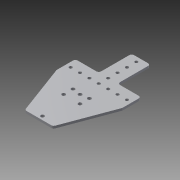
# Autodesk Inventor part: Roller Pneumatic Back Connector (Custom)
Saved by Autodesk Inventor 2014 (Build 180170000, 170)
## iProperties
Created: 2014-01-06
Part Number: Roller Pneumatic Back Connector (Custom)
Material: Aluminum 6061
Document SubType Name: Modeling
Designer: Andrew Toennies
Density: 2.71 g/cm^3
Appearance: Aluminum - Flat
Mass: 64.1686 g
Surface Area: 169.384 cm^2
Volume: 23.6785 cm^3
Author: Andrew Toennies
Autodesk Inventor part; units mm, degrees
ref_plane "YZ Plane" through (0, 0, 0) normal (1, 0, 0) x (0, 1, 0)
ref_plane "XZ Plane" through (0, 0, 0) normal (0, 1, 0) x (-1, 0, 0)
ref_plane "XY Plane" through (0, 0, 0) normal (0, 0, 1) x (1, 0, 0)
sketch "Sketch1" plane through (0, 0, 0) normal (0, 1, 0) x (-1, 0, 0)
  circle A0 centre (0, 0) radius 2.413
  circle A1 centre (0, 50.8) radius 2.413
  line L0 (0, 50.8) -> (0, 0) construction
  circle A2 centre (11.049, 11.1125) radius 2.413
  circle A3 centre (11.049, -1.5875) radius 2.413
  circle A4 centre (-11.049, -1.5875) radius 2.413
  circle A5 centre (-11.049, 11.1125) radius 2.413
  line L1 (-11.049, -1.5875) -> (-11.049, 11.1125) construction
  line L2 (-11.049, 11.1125) -> (11.049, 11.1125) construction
  line L3 (19.05, 55.5625) -> (-19.05, 55.5625)
  line L4 (-44.45, -12.7) -> (-44.45, -38.1)
  line L5 (-44.45, -38.1) -> (-15.875, -38.1)
  line L6 (-12.7, -41.275) -> (-12.7, -82.55)
  line L7 (-12.7, -82.55) -> (12.7, -82.55)
  line L8 (12.7, -82.55) -> (12.7, -41.275)
  line L9 (15.875, -38.1) -> (44.45, -38.1)
  line L10 (44.45, -38.1) -> (44.45, -12.7)
  line L11 (44.45, -12.7) -> (19.05, 55.5625)
  line L12 (-44.45, -12.7) -> (-19.05, 55.5625)
  circle A6 centre (-38.1, -25.4) radius 2.0701
  circle A7 centre (-25.4, -25.4) radius 2.0701
  circle A8 centre (-12.7, -25.4) radius 2.0701
  circle A9 centre (0, -25.4) radius 2.0701
  circle A10 centre (12.7, -25.4) radius 2.0701
  circle A11 centre (25.4, -25.4) radius 2.0701
  circle A12 centre (38.1, -25.4) radius 2.0701
  arc A13 (-12.7, -41.275) -> (-15.875, -38.1) centre (-15.875, -41.275) ccw
  arc A14 (15.875, -38.1) -> (12.7, -41.275) centre (15.875, -41.275) ccw
  circle A15 centre (0, -76.2) radius 2.0701
  circle A16 centre (0, -63.5) radius 2.0701
  circle A17 centre (0, -50.8) radius 2.0701
  circle A18 centre (0, -38.1) radius 2.0701
  point P0 (0, 25.4)
  point P1 (-12.7, -38.1)
  point P2 (12.7, -38.1)
  dimension "d1" = 4.826
  dimension "d2" = 50.8
  dimension "d3" = 4.826
  dimension "d4" = 4.826
  dimension "d5" = 12.7
  dimension "d6" = 11.049
  dimension "d7" = 11.049
  dimension "d9" = 4.826
  dimension "d10" = 4.826
  dimension "d11" = 11.049
  dimension "d12" = 12.7
  dimension "d23" = 1.5875
  dimension "d24" = 31.75
  dimension "d25" = 44.45
  dimension "d26" = 25.4
  dimension "d28" = 44.45
  dimension "d29" = 38.1
  dimension "d30" = 38.1
  dimension "d31" = 19.05
  dimension "d32" = 68.2625
  dimension "d33" = 4.1402
  dimension "d34" = 12.7
  dimension "d35" = 6.35
  dimension "d38" = 12.7
  dimension "d43" = 3.175
  dimension "d44" = 4.1402
  dimension "d45" = 6.35
  dimension "d46" = 12.7
  dimension "d49" = 12.7
  constraints: 26 end point, 19 centre point, 6 perpendicular, 4 equal length, 4 point on circle, 4 point on line, 4 tangent, 3 parallel, 3 vertical, 2 equal radius, 1 coincident, 1 horizontal, 1 midpoint, 18 other
  measures "d1" diameter of A1
  measures "d2" distance of L0.start L0.end
  measures "d3" diameter of A2
  measures "d4" diameter of A3
  measures "d5" distance of A3.centre L2.end
  measures "d6" distance from line of L0 A3.centre
  measures "d7" distance from line of L0 L2.end
  measures "d9" diameter of A4
  measures "d10" diameter of A5
  measures "d11" distance between parallel lines of L1 L0
  measures "d12" distance of L1.start L1.end
  measures "d23" vertical distance of A3.centre L0.end
  measures "d24" distance of L4.end point (-12.7, -38.1)
  measures "d25" distance of point (-12.7, -38.1) L6.end
  measures "d26" distance of L6.end L7.end
  measures "d28" distance from line of L4 point (0, 0)
  measures "d29" distance from line of L5 point (0, 0)
  measures "d30" distance of L3.start L3.end
  measures "d31" horizontal distance of point (0, 0) L3.end
  measures "d32" distance from line of L4.start L3
  measures "d33" diameter of A6
  measures "d34" distance from line of L5 A6.centre
  measures "d35" distance from line of L4 A6.centre
  measures "d38" distance of A6.centre A7.centre
  measures "d43" radius of A13
  measures "d44" diameter of A15
  measures "d45" distance from line of L7 A15.centre
  measures "d46" distance from line of L6 A15.centre
  measures "d49" distance of A15.centre A16.centre
extrude "Extrusion1" add sketch "Sketch1" along normal blind 3.175
fillet "Fillet1" radius 3.175 2 edges at (19.05, 1.5875, 55.5625) (-19.05, 1.5875, 55.5625)
fillet "Fillet2" radius 3.175 6 edges at (44.45, 1.5875, -38.1) (12.7, 1.5875, -82.55) (-12.7, 1.5875, -82.55) (-44.45, 1.5875, -38.1) (-44.45, 1.5875, -12.7) (44.45, 1.5875, -12.7)
equation "\"d7\" = d6"
equation "\"d11\" = d6"
body "Solid1"
